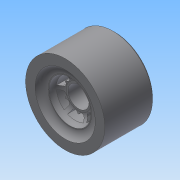
# Autodesk Inventor part: Wheels
Saved by Autodesk Inventor 2015 (Build 190159000, 159)
## iProperties
Created: 2016-01-06
Part Number: Wheels
Material: Generic
Document SubType Name: Modeling
Designer: JoshuaYuan
Density: 1 g/cm^3
Appearance: Default
Author: JoshuaYuan
Autodesk Inventor part; units mm, degrees
ref_plane "YZ Plane" through (0, 0, 0) normal (1, 0, 0) x (0, 1, 0)
ref_plane "XZ Plane" through (0, 0, 0) normal (0, 1, 0) x (-1, 0, 0)
ref_plane "XY Plane" through (0, 0, 0) normal (0, 0, 1) x (1, 0, 0)
sketch "Sketch1" plane through (0, 0, 0) normal (0, 0, 1) x (1, 0, 0)
  line L0 (-58.1, 0) -> (58.1, 0) projected
  line L1 (0, -58.1) -> (0, 58.1) projected
  circle A0 centre (0, 0) radius 41.5
  circle A1 centre (0, 0) radius 31.5
  circle A2 centre (0, 0) radius 22
  circle A3 centre (0, 0) radius 11
  circle A4 centre (0, 0) radius 4
  dimension "d0" = 83
  dimension "d1" = 10
  dimension "d2" = 8
  dimension "d3" = 22
  dimension "d11" = 44
  constraints: 5 centre point, 5 coincident
  measures "d0" diameter of A0
  measures "d1" radial gap between concentric circles of A0 A1
  measures "d2" diameter of A4
  measures "d3" diameter of A3
  measures "d11" diameter of A2
extrude "Outside" add sketch "Sketch1" along normal mid plane 52 contours A1 L1 A0 L0 | L0 A0 L1 A1 | A1 L0 A0 L1 | L1 A0 L0 A1
extrude "Middle" add sketch "Sketch1" along normal mid plane 42 contours A2 L1 A1 L0 | L0 A1 L1 A2 | A2 L0 A1 L1 | L1 A1 L0 A2
extrude "Inside" add sketch "Sketch1" along normal mid plane 24 contours A3 L1 A2 L0 | L0 A2 L1 A3 | A3 L0 A2 L1 | L1 A2 L0 A3
fillet "outside-outer fillet" radius 10 1 edges at (-31.5, 0, 21)
sketch "spokes" plane through (0, 0, 12) normal (0, 0, 1) x (1, 0, 0)
  arc A0 (11.6992, -16.2216) -> (19.9001, -2) centre (0, 0) ccw
  line L0 (11.6992, -16.2216) -> (9.7171, -12.7886)
  line L1 (19.9001, -2) -> (15.9359, -2)
  arc A1 (15.9359, -2) -> (13.6483, -7.064) centre (15.9359, -5.0487) ccw
  arc A2 (12.9527, -8.2707) -> (9.7171, -12.7886) centre (12.3551, -11.2603) ccw
  circle A3 centre (0, 0) radius 22 projected
  arc A4 (12.9527, -8.2707) -> (13.6483, -7.064) centre (0, 0) ccw
  circle A5 centre (0, 0) radius 11 projected
  line L2 (-58.1, 0) -> (58.1, 0) projected
  arc A6 (19.8979, 2.021) -> (11.6821, 16.234) centre (0, 0) ccw
  line L3 (19.8979, 2.021) -> (15.9338, 2.021)
  line L4 (11.6821, 16.234) -> (9.7, 12.8009)
  arc A7 (9.7, 12.8009) -> (12.9418, 8.2877) centre (12.3403, 11.2765) ccw
  arc A8 (13.639, 7.082) -> (15.9338, 2.021) centre (15.9292, 5.0697) ccw
  arc A9 (13.639, 7.082) -> (12.9418, 8.2877) centre (0, 0) ccw
  arc A10 (8.1987, 18.2426) -> (-8.218, 18.234) centre (0, 0) ccw
  line L5 (8.1987, 18.2426) -> (6.2167, 14.8095)
  line L6 (-8.218, 18.234) -> (-6.2359, 14.8009)
  arc A11 (-6.2359, 14.8009) -> (-0.7065, 15.3518) centre (-3.5956, 16.3252) ccw
  arc A12 (0.6863, 15.3527) -> (6.2167, 14.8095) centre (3.5741, 16.33) ccw
  arc A13 (0.6863, 15.3527) -> (-0.7065, 15.3518) centre (0, 0) ccw
  arc A14 (-11.6992, 16.2216) -> (-19.9001, 2) centre (0, 0) ccw
  line L7 (-11.6992, 16.2216) -> (-9.7171, 12.7886)
  line L8 (-19.9001, 2) -> (-15.9359, 2)
  arc A15 (-15.9359, 2) -> (-13.6483, 7.064) centre (-15.9359, 5.0487) ccw
  arc A16 (-12.9527, 8.2707) -> (-9.7171, 12.7886) centre (-12.3551, 11.2603) ccw
  arc A17 (-12.9527, 8.2707) -> (-13.6483, 7.064) centre (0, 0) ccw
  arc A18 (-19.8979, -2.021) -> (-11.6821, -16.234) centre (0, 0) ccw
  line L9 (-19.8979, -2.021) -> (-15.9338, -2.021)
  line L10 (-11.6821, -16.234) -> (-9.7, -12.8009)
  arc A19 (-9.7, -12.8009) -> (-12.9418, -8.2877) centre (-12.3403, -11.2765) ccw
  arc A20 (-13.639, -7.082) -> (-15.9338, -2.021) centre (-15.9292, -5.0697) ccw
  arc A21 (-13.639, -7.082) -> (-12.9418, -8.2877) centre (0, 0) ccw
  arc A22 (-8.1987, -18.2426) -> (8.218, -18.234) centre (0, 0) ccw
  line L11 (-8.1987, -18.2426) -> (-6.2167, -14.8095)
  line L12 (8.218, -18.234) -> (6.2359, -14.8009)
  arc A23 (6.2359, -14.8009) -> (0.7065, -15.3518) centre (3.5956, -16.3252) ccw
  arc A24 (-0.6863, -15.3527) -> (-6.2167, -14.8095) centre (-3.5741, -16.33) ccw
  arc A25 (-0.6863, -15.3527) -> (0.7065, -15.3518) centre (0, 0) ccw
  circle A26 centre (0, 0) radius 12.601
  circle A27 centre (0, 0) radius 16.7165 construction
  dimension "d14" = 60
  dimension "d17" = 360
  dimension "d23" = 2
  constraints: 50 point on circle, 26 centre point, 24 end point, 4 coincident, 2 concentric, 1 equal length, 1 equal radius, 1 parallel, 1 tangent, 113 other
  measures "d14" angle of L1 L0
  measures "d23" distance between parallel lines of L2 L1
fillet "outside-spoke fillet" radius 9 1 edges at (-22, 0, 12)
chamfer "inside-edge chamfer" distance 2 angle 45 1 edges at (-41.5, 0, -26)
fillet "inside-outer fillet" radius 11 1 edges at (-31.5, 0, -21)
fillet "inside-spoke fillet" radius 9 1 edges at (-22, 0, -12)
extrude "spoke cutouts" cut sketch "spokes" along normal through all both and the other way through all contours L0 A2 A4 A1 L1 A0 | L3 A8 A9 A7 L4 A6 | L5 A12 A13 A11 L6 A10 | L7 A16 A17 A15 L8 A14 | L9 A20 A21 A19 L10 A18 | L11 A24 A25 A23 L12 A22
body "Solid1"
